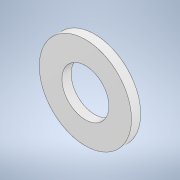
# Autodesk Inventor part: TT-1020-20
Saved by Autodesk Inventor 2020.4 (Build 244396000, 396)
## iProperties
Part Number: TT-1020-20
Material: PET プラスチック
Document SubType Name: Modeling
Designer: Masato Kubotera
Density: 2.13737 g/cm^3
Appearance: 滑らか - 白
Mass: 0.99365 g
Surface Area: 6.54645 cm^2
Volume: 0.464893 cm^3
Description: ReadyMade
Catalog Web Link: https://www.hirosugi-net.co.jp/shop/g/g31941/
Author: Masato Kubotera
Autodesk Inventor part; units mm, degrees
ref_plane "YZ Plane" through (0, 0, 0) normal (1, 0, 0) x (0, 1, 0)
ref_plane "XZ Plane" through (0, 0, 0) normal (0, 1, 0) x (-1, 0, 0)
ref_plane "XY Plane" through (0, 0, 0) normal (0, 0, 1) x (1, 0, 0)
sketch "スケッチ1" plane through (0, 0, 0) normal (0, 0, 1) x (1, 0, 0)
  circle A0 centre (0, 0) radius 5.1
  circle A1 centre (0, 0) radius 10
  dimension "d0" = 10.2
  dimension "d1" = 20
  constraints: 2 centre point, 2 coincident
  measures "d0" diameter of A0
  measures "d1" diameter of A1
extrude "押し出し1" add sketch "スケッチ1" along normal blind 2
